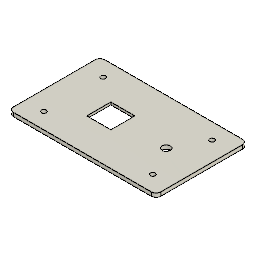
ScaleFaceplate (Autodesk Fusion 360 design; units mm, degrees)
Autodesk Fusion 360 part; units mm, degrees
sketch "Sketch1" plane through (0, 0, 0) normal (0, 0, 1) x (1, 0, 0)
  line L0 (3.81, 0) -> (113.03, 0)
  line L1 (116.84, 3.81) -> (116.84, 68.58)
  line L2 (113.03, 72.39) -> (3.81, 72.39)
  line L3 (0, 68.58) -> (0, 3.81)
  arc A0 (0, 3.81) -> (3.81, 0) centre (3.81, 3.81) ccw
  arc A1 (113.03, 0) -> (116.84, 3.81) centre (113.03, 3.81) ccw
  arc A2 (116.84, 68.58) -> (113.03, 72.39) centre (113.03, 68.58) ccw
  arc A3 (3.81, 72.39) -> (0, 68.58) centre (3.81, 68.58) ccw
  circle A4 centre (15.24, 12.7) radius 1.905
  circle A5 centre (101.6, 12.7) radius 1.905
  circle A6 centre (101.6, 59.69) radius 1.905
  circle A7 centre (15.24, 59.69) radius 1.905
  point P0 (116.84, 0)
  point P1 (0, 72.39)
  dimension "d1" = 116.84
  dimension "d2" = 72.39
  dimension "d3" = 3.81
  dimension "d4" = 3.81
  dimension "d5" = 3.81
  dimension "d6" = 3.81
  dimension "d7" = 3.81
  dimension "d8" = 15.24
  dimension "d9" = 12.7
  dimension "d10" = 3.81
  dimension "d11" = 3.81
  dimension "d12" = 3.81
  constraint horizontal L0
  constraint vertical L1
  constraint horizontal L2
  constraint vertical L3
  constraint coincident origin L3
  constraint coincident origin L0
  constraint tangent L3 A0
  constraint tangent L0 A0
  constraint coincident P0 L0
  constraint coincident P0 L1
  constraint tangent L0 A1
  constraint tangent L1 A1
  constraint tangent L2 A2
  constraint tangent L1 A2
  constraint coincident P1 L3
  constraint coincident P1 L2
  constraint tangent L3 A3
  constraint tangent L2 A3
  measures "d1" distance of origin P0
  measures "d2" distance of origin P1
  measures "d3" radius of A0
  measures "d4" radius of A1
  measures "d5" radius of A2
  measures "d6" radius of A3
  measures "d7" diameter of A4
  measures "d8" distance of L3 A4.centre
  measures "d9" distance of L0 A4.centre
  measures "d10" diameter of A5
  measures "d11" diameter of A6
  measures "d12" diameter of A7
extrude "Extrude1" add sketch "Sketch1" along normal blind 3.048
sketch "Sketch2" plane through (0, 0, 0) normal (0, 0, -1) x (1, 0, 0)
  circle A0 centre (15.24, -59.69) radius 1.905
  circle A1 centre (101.6, -59.69) radius 1.905
  circle A2 centre (15.24, -12.7) radius 1.905
  circle A3 centre (101.6, -12.7) radius 1.905
  arc A4 (0, -68.58) -> (3.81, -72.39) centre (3.81, -68.58) ccw
  line L0 (3.81, -72.39) -> (113.03, -72.39)
  arc A5 (113.03, -72.39) -> (116.84, -68.58) centre (113.03, -68.58) ccw
  line L1 (116.84, -68.58) -> (116.84, -3.81)
  arc A6 (116.84, -3.81) -> (113.03, 0) centre (113.03, -3.81) ccw
  line L2 (113.03, 0) -> (3.81, 0)
  arc A7 (3.81, 0) -> (0, -3.81) centre (3.81, -3.81) ccw
  line L3 (0, -3.81) -> (0, -68.58)
  line L4 (34.29, -22.695) -> (64.77, -22.695)
  line L5 (64.77, -22.695) -> (64.77, -49.695)
  line L6 (64.77, -49.695) -> (34.29, -49.695)
  line L7 (34.29, -49.695) -> (34.29, -22.695)
  circle A8 centre (88.9518, -36.0108) radius 3.175
  line L8 (0, -36.195) -> (116.84, -36.195) construction
  line L9 (35.306, -26.695) -> (54.306, -26.695)
  line L10 (54.306, -26.695) -> (54.306, -45.695)
  line L11 (54.306, -45.695) -> (35.306, -45.695)
  line L12 (35.306, -45.695) -> (35.306, -26.695)
  line L13 (35.306, -26.695) -> (54.306, -45.695) construction
  line L14 (54.306, -26.695) -> (35.306, -45.695) construction
  circle A9 centre (35.814, -24.765) radius 1.016
  circle A10 centre (38.354, -24.765) radius 1.016
  circle A11 centre (40.894, -24.765) radius 1.016
  circle A12 centre (43.434, -24.765) radius 1.016
  circle A13 centre (45.974, -24.765) radius 1.016
  circle A14 centre (48.514, -24.765) radius 1.016
  circle A15 centre (51.054, -24.765) radius 1.016
  circle A16 centre (53.594, -24.765) radius 1.016
  circle A17 centre (35.814, -47.625) radius 1.016
  circle A18 centre (38.354, -47.625) radius 1.016
  circle A19 centre (40.894, -47.625) radius 1.016
  circle A20 centre (43.434, -47.625) radius 1.016
  circle A21 centre (45.974, -47.625) radius 1.016
  circle A22 centre (48.514, -47.625) radius 1.016
  circle A23 centre (51.054, -47.625) radius 1.016
  circle A24 centre (53.594, -47.625) radius 1.016
  point P0 (44.806, -36.195)
  dimension "d15" = 30.48
  dimension "d16" = 27
  dimension "d18" = 34.29
  dimension "d19" = 6.35
  dimension "d20" = 19
  dimension "d21" = 19
  dimension "d22" = 1.016
  dimension "d23" = 2.032
  dimension "d26" = 2.54
  dimension "d27" = -22.86
  dimension "d29" = 1.524
  dimension "d37" = 11.43
  constraint horizontal L4
  constraint vertical L5
  constraint horizontal L6
  constraint vertical L7
  constraint midpoint L3 L8.start
  constraint midpoint L1 L8.end
  constraint perpendicular L9 L10
  constraint parallel L9 L11
  constraint parallel L10 L12
  constraint horizontal L9
  constraint coincident L13 P0
  constraint coincident L14 P0
  constraint coincident L8 P0
  constraint symmetric L4 L6 L8
  measures "d15" distance of L4.start L4.end
  measures "d16" distance of L4.start L6.end
  measures "d18" distance of L3 L7
  measures "d19" diameter of A8
  measures "d20" distance of L9.end L10.end
  measures "d21" distance of L10.end L11.end
  measures "d22" distance of L7 L12
  measures "d23" diameter of A9
  measures "d29" distance of L7 A9.centre
  measures "d37" distance of L8 A9.centre
extrude "Extrude2" cut sketch "Sketch2" against normal through all contours L9 L10 L11 L12
extrude "Extrude3" cut sketch "Sketch2" against normal blind 2.032 contours A9 | A10 | A11 | A12 | A13 | A14 | A15 | A16 | A17 | A18 | A19 | A20 | A21 | A22 | A23 | A24
extrude "Extrude4" cut sketch "Sketch2" against normal blind 1.016 contours L4 L5 L6 L7
extrude "Extrude5" cut sketch "Sketch2" against normal through all contours A8
